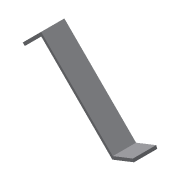
# Autodesk Inventor part: LoadSlideBracket
Saved by Autodesk Inventor 2015 (Build 190159000, 159)
## iProperties
Created: 2015-03-06
Part Number: LoadSlideBracket
Material: Generic
Document SubType Name: Modeling
Designer: Jaden
Density: 1 g/cm^3
Appearance: Default
Author: Jaden
Autodesk Inventor part; units mm, degrees
ref_plane "YZ Plane" through (0, 0, 0) normal (1, 0, 0) x (0, 1, 0)
ref_plane "XZ Plane" through (0, 0, 0) normal (0, 1, 0) x (-1, 0, 0)
ref_plane "XY Plane" through (0, 0, 0) normal (0, 0, 1) x (1, 0, 0)
sketch "Sketch1" plane through (0, 0, 0) normal (0, 0, 1) x (1, 0, 0)
  line L0 (0, 0) -> (17.9605, 17.9605)
  line L1 (0, 0) -> (25.4, 0) construction
  line L2 (17.7799, 22.2704) -> (-2.2453, 2.2453)
  line L3 (-2.2453, 2.2453) -> (0, 0)
  line L4 (17.9605, 17.9605) -> (95.5858, -59.6648)
  line L5 (17.9605, 17.9605) -> (127.7393, 17.9605) construction
  line L6 (95.5858, -59.6648) -> (119.2185, -50.3557)
  line L7 (95.5858, -59.6648) -> (120.9858, -59.6648) construction
  line L8 (119.2185, -50.3557) -> (118.0548, -47.4016)
  line L9 (118.0548, -47.4016) -> (96.1001, -56.0498)
  line L10 (96.1001, -56.0498) -> (17.7799, 22.2704)
  dimension "d14" = 25.4
  dimension "d15" = 45
  dimension "d24" = 109.7788
  dimension "d25" = 45
  dimension "d26" = 25.4
  dimension "d27" = 21.5
  dimension "d28" = 3.175
  dimension "d29" = 23.5966
  constraints: 22 end point, 3 equal length, 3 horizontal, 3 perpendicular
  measures "d14" distance of L0.start L0.end
  measures "d15" angle of L1 L0
  measures "d24" distance of L0.end L4.end
  measures "d25" angle of L4 L5
  measures "d26" distance of L4.end L6.end
  measures "d27" angle of L7 L6
  measures "d28" distance of L6.end L8.end
  measures "d29" distance of L8.end L9.end
extrude "Extrusion2" add sketch "Sketch1" along normal blind 25.4
body "Solid2"
